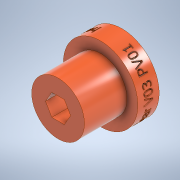
# Autodesk Inventor part: hexBushingForSideWormGear
Saved by Autodesk Inventor 2022.2 (Build 262287010, 287A)
## iProperties
Created: 2020-11-16
Part Number: hexBushingForSideWormGear
Material: PC/ABS Plastic
Document SubType Name: Modeling
Designer: robst
Density: 0.357273 g/cm^3
Appearance: Smooth - Light Orange
Author: robst
Autodesk Inventor part; units mm, degrees
ref_plane "YZ Plane" through (0, 0, 0) normal (1, 0, 0) x (0, 1, 0)
ref_plane "XY Plane" through (0, 0, 0) normal (0, 0, 1) x (1, 0, 0)
sketch "Sketch1" plane through (0, 0, 0) normal (0, 0, 1) x (1, 0, 0)
  line L0 (7.3323, 0) -> (3.6662, -6.35)
  line L1 (3.6662, -6.35) -> (-3.6662, -6.35)
  line L2 (-3.6662, -6.35) -> (-7.3323, 0)
  line L3 (-7.3323, 0) -> (-3.6662, 6.35)
  line L4 (-3.6662, 6.35) -> (3.6662, 6.35)
  line L5 (3.6662, 6.35) -> (7.3323, 0)
  point P0 (0, 0)
  point P1 (0, 0)
  dimension "d0" = 12.7
  constraints: 12 end point, 1 coincident, 1 horizontal, 13 other
  measures "d0" distance between parallel lines of L1 L4
extrude "Extrusion1" add sketch "Sketch1" along normal mid plane 25.4
sketch "Sketch2" plane through (0, 0, -12.7) normal (0, 0, -1) x (-1, 0, 0)
  circle A0 centre (0, 0) radius 15.748
  dimension "d3" = 31.496
  constraints: 1 centre point, 1 coincident
  measures "d3" diameter of A0
extrude "Extrusion2" add sketch "Sketch2" along normal blind 19.05
sketch "Sketch3" plane through (0, 0, -31.75) normal (0, 0, -1) x (-1, 0, 0)
  circle A0 centre (0, 0) radius 22.225
  dimension "d6" = 44.45
  constraints: 1 centre point, 1 coincident
  measures "d6" diameter of A0
extrude "Base" add sketch "Sketch3" along normal blind 12.7
sketch "Sketch6" plane through (-3.6662, 6.35, 12.7) normal (0, 1, 0) x (1, 0, 0)
  line L0 (7.3323, 0) -> (0, 0) construction
  line L1 (3.6662, 0) -> (3.6662, 34.6111) construction
  line L2 (19.4142, 25.4) -> (-12.0818, 25.4) projected
  point P0 (3.6662, 12.7)
  point P1 (3.6662, 19.2024)
  dimension "d13" = 6.1976
  constraints: 2 end point, 1 midpoint, 1 point on line, 1 vertical
  measures "d13" distance from line of point (3.666, 19.202) L2
hole "Hole1" at (0, 6.35, -6.5024) direction (0, -1, 0) diameter 4.318 end through all clearance for "Hex Machine Screw" size "#6" standard "Ansi Unified Screw Threads"
sketch "Sketch7" plane through (0, 0, 12.7) normal (0, 0, 1) x (1, 0, 0)
  point P0 (0, 0)
  point P1 (0, 0)
  constraints: 1 coincident
hole "Hole2" at (0, 0, 12.7) direction (0, 0, -1) diameter 6.3246 depth 7.874 counterbore diameter 6.604 counterbore depth 6.1239
ref_plane "Work Plane1" through (0, -22.225, -31.75) normal (0, 1, 0) x (-1, 0, 0)
sketch "Sketch8" plane through (0, -22.225, -31.75) normal (0, 1, 0) x (-1, 0, 0)
  line L0 (-22.225, -12.7) -> (22.225, -12.7) projected
  line L1 (-22.225, 0) -> (22.225, 0) projected
  line L2 (22.225, 0) -> (22.225, -12.7) construction
  line L3 (22.225, -6.35) -> (-22.225, -6.35) construction
  line L4 (-22.225, 0) -> (-22.225, -12.7) construction
  line L5 (58.138, -8.89) -> (58.7802, -8.89)
  line L6 (58.7802, -8.89) -> (58.7802, -6.7164)
  spline S0 degree 2 poles (58.7802, -6.7164) (58.7802, -6.4529) (58.8296, -6.0001) (58.9037, -5.8642) knots 0 0 0 1 2 2 2
  spline S1 degree 2 poles (58.9037, -5.8642) (58.9819, -5.7201) (59.2619, -5.5802) (59.5006, -5.5802) knots 0 0 0 1 2 2 2
  spline S2 degree 2 poles (59.5006, -5.5802) (59.7394, -5.5802) (60.2458, -5.8354) (60.4886, -6.0412) knots 0 0 0 1 2 2 2
  line L7 (60.4886, -6.0412) -> (60.4886, -8.89)
  line L8 (60.4886, -8.89) -> (61.1308, -8.89)
  line L9 (61.1308, -8.89) -> (61.1308, -3.5836)
  line L10 (61.1308, -3.5836) -> (60.4886, -3.5836)
  line L11 (60.4886, -3.5836) -> (60.4886, -5.502)
  spline S3 degree 2 poles (60.4886, -5.502) (60.2005, -5.2426) (59.6447, -4.9709) (59.3318, -4.9709) knots 0 0 0 1 2 2 2
  spline S4 degree 2 poles (59.3318, -4.9709) (58.772, -4.9709) (58.138, -5.7119) (58.138, -6.4159) knots 0 0 0 1 2 2 2
  line L12 (58.138, -6.4159) -> (58.138, -8.89)
  spline S5 degree 2 poles (55.5815, -8.9765) (56.4954, -8.9765) (57.4999, -7.9514) (57.4999, -7.0046) knots 0 0 0 1 2 2 2
  spline S6 degree 2 poles (57.4999, -7.0046) (57.4999, -6.0742) (56.5243, -4.9709) (55.738, -4.9709) knots 0 0 0 1 2 2 2
  spline S7 degree 2 poles (55.738, -4.9709) (55.3839, -4.9709) (54.8364, -5.1767) (54.6347, -5.3949) knots 0 0 0 1 2 2 2
  spline S8 degree 2 poles (54.6347, -5.3949) (54.4289, -5.6131) (54.2107, -6.243) (54.2107, -6.6999) knots 0 0 0 1 2 2 2
  line L13 (54.2107, -6.6999) -> (54.2107, -7.0498)
  line L14 (54.2107, -7.0498) -> (56.8495, -7.0498)
  spline S9 degree 2 poles (56.8495, -7.0498) (56.8495, -7.7126) (56.1826, -8.4166) (55.5898, -8.4166) knots 0 0 0 1 2 2 2
  spline S10 degree 2 poles (55.5898, -8.4166) (55.3798, -8.4166) (54.9723, -8.3219) (54.8076, -8.2478) knots 0 0 0 1 2 2 2
  spline S11 degree 2 poles (54.8076, -8.2478) (54.6347, -8.1655) (54.3959, -8.0214) (54.3177, -7.9555) knots 0 0 0 1 2 2 2
  line L15 (54.3177, -7.9555) -> (54.2807, -7.9555)
  line L16 (54.2807, -7.9555) -> (54.2807, -8.6553)
  spline S12 degree 2 poles (54.2807, -8.6553) (54.3918, -8.7006) (54.7294, -8.8324) (54.8611, -8.8694) knots 0 0 0 1 2 2 2
  spline S13 degree 2 poles (54.8611, -8.8694) (55.0464, -8.9229) (55.351, -8.9765) (55.5815, -8.9765) knots 0 0 0 1 2 2 2
  spline S14 degree 2 poles (54.8364, -6.56) (54.8447, -6.3006) (54.9517, -5.9219) (55.0546, -5.7942) knots 0 0 0 1 2 2 2
  spline S15 degree 2 poles (55.0546, -5.7942) (55.1658, -5.6502) (55.5157, -5.4978) (55.775, -5.4978) knots 0 0 0 1 2 2 2
  spline S16 degree 2 poles (55.775, -5.4978) (56.0303, -5.4978) (56.3884, -5.6502) (56.5366, -5.7984) knots 0 0 0 1 2 2 2
  spline S17 degree 2 poles (56.5366, -5.7984) (56.6807, -5.9507) (56.8289, -6.3171) (56.8495, -6.56) knots 0 0 0 1 2 2 2
  line L17 (56.8495, -6.56) -> (54.8364, -6.56)
  line L18 (50.6003, -8.89) -> (51.3866, -8.89)
  line L19 (51.3866, -8.89) -> (52.3129, -7.4574)
  line L20 (52.3129, -7.4574) -> (53.2638, -8.89)
  line L21 (53.2638, -8.89) -> (53.9925, -8.89)
  line L22 (53.9925, -8.89) -> (52.671, -7.0004)
  line L23 (52.671, -7.0004) -> (53.9801, -5.0779)
  line L24 (53.9801, -5.0779) -> (53.1939, -5.0779)
  line L25 (53.1939, -5.0779) -> (52.2717, -6.4982)
  line L26 (52.2717, -6.4982) -> (51.329, -5.0779)
  line L27 (51.329, -5.0779) -> (50.6003, -5.0779)
  line L28 (50.6003, -5.0779) -> (51.9136, -6.9593)
  line L29 (51.9136, -6.9593) -> (50.6003, -8.89)
  spline S18 degree 2 poles (46.6071, -7.3298) (46.6071, -7.7085) (46.8953, -8.289) (47.1341, -8.4783) knots 0 0 0 1 2 2 2
  spline S19 degree 2 poles (47.1341, -8.4783) (47.4223, -8.7006) (48.0768, -8.89) (48.5955, -8.89) knots 0 0 0 1 2 2 2
  line L30 (48.5955, -8.89) -> (50.0528, -8.89)
  line L31 (50.0528, -8.89) -> (50.0528, -3.81)
  line L32 (50.0528, -3.81) -> (48.7067, -3.81)
  spline S20 degree 2 poles (48.7067, -3.81) (48.1633, -3.81) (47.6199, -3.88) (47.3729, -4.0158) knots 0 0 0 1 2 2 2
  spline S21 degree 2 poles (47.3729, -4.0158) (47.097, -4.1599) (46.8459, -4.6333) (46.8459, -4.9544) knots 0 0 0 1 2 2 2
  spline S22 degree 2 poles (46.8459, -4.9544) (46.8459, -5.3126) (47.2247, -5.8807) (47.5581, -6.0412) knots 0 0 0 1 2 2 2
  line L33 (47.5581, -6.0412) -> (47.5581, -6.0659)
  spline S23 degree 2 poles (47.5581, -6.0659) (47.1053, -6.1894) (46.6071, -6.844) (46.6071, -7.3298) knots 0 0 0 1 2 2 2
  spline S24 degree 2 poles (47.3111, -7.3586) (47.3111, -7.0704) (47.4758, -6.6999) (47.7228, -6.5682) knots 0 0 0 1 2 2 2
  spline S25 degree 2 poles (47.7228, -6.5682) (47.8833, -6.4859) (48.2621, -6.4365) (48.612, -6.4365) knots 0 0 0 1 2 2 2
  line L34 (48.612, -6.4365) -> (49.3777, -6.4365)
  line L35 (49.3777, -6.4365) -> (49.3777, -8.3137)
  line L36 (49.3777, -8.3137) -> (48.8302, -8.3137)
  spline S26 degree 2 poles (48.8302, -8.3137) (48.3856, -8.3137) (47.8751, -8.2313) (47.6775, -8.0996) knots 0 0 0 1 2 2 2
  spline S27 degree 2 poles (47.6775, -8.0996) (47.4881, -7.9637) (47.3111, -7.6262) (47.3111, -7.3586) knots 0 0 0 1 2 2 2
  spline S28 degree 2 poles (47.5499, -5.0491) (47.5499, -4.868) (47.6734, -4.5963) (47.8092, -4.5181) knots 0 0 0 1 2 2 2
  spline S29 degree 2 poles (47.8092, -4.5181) (47.9739, -4.4275) (48.3732, -4.3863) (48.7314, -4.3863) knots 0 0 0 1 2 2 2
  line L37 (48.7314, -4.3863) -> (49.3777, -4.3863)
  line L38 (49.3777, -4.3863) -> (49.3777, -5.8725)
  line L39 (49.3777, -5.8725) -> (48.612, -5.8725)
  spline S30 degree 2 poles (48.612, -5.8725) (48.295, -5.8725) (47.9945, -5.8066) (47.8339, -5.7037) knots 0 0 0 1 2 2 2
  spline S31 degree 2 poles (47.8339, -5.7037) (47.6775, -5.6049) (47.5499, -5.2879) (47.5499, -5.0491) knots 0 0 0 1 2 2 2
  line L40 (43.0215, -8.89) -> (43.6637, -8.89)
  line L41 (43.6637, -8.89) -> (43.6637, -8.4701)
  spline S32 degree 2 poles (43.6637, -8.4701) (43.9601, -8.7294) (44.4912, -8.997) (44.8205, -8.997) knots 0 0 0 1 2 2 2
  spline S33 degree 2 poles (44.8205, -8.997) (45.0675, -8.997) (45.508, -8.8324) (45.6685, -8.6553) knots 0 0 0 1 2 2 2
  spline S34 degree 2 poles (45.6685, -8.6553) (45.8332, -8.4783) (46.0143, -7.939) (46.0143, -7.5521) knots 0 0 0 1 2 2 2
  line L42 (46.0143, -7.5521) -> (46.0143, -5.0779)
  line L43 (46.0143, -5.0779) -> (45.3721, -5.0779)
  line L44 (45.3721, -5.0779) -> (45.3721, -7.2516)
  spline S35 degree 2 poles (45.3721, -7.2516) (45.3721, -7.5562) (45.3269, -7.9555) (45.2486, -8.1037) knots 0 0 0 1 2 2 2
  spline S36 degree 2 poles (45.2486, -8.1037) (45.1704, -8.2519) (44.9028, -8.3878) (44.6517, -8.3878) knots 0 0 0 1 2 2 2
  spline S37 degree 2 poles (44.6517, -8.3878) (44.4171, -8.3878) (43.886, -8.1202) (43.6637, -7.9267) knots 0 0 0 1 2 2 2
  line L45 (43.6637, -7.9267) -> (43.6637, -5.0779)
  line L46 (43.6637, -5.0779) -> (43.0215, -5.0779)
  line L47 (43.0215, -5.0779) -> (43.0215, -8.89)
  spline S38 degree 2 poles (41.062, -8.9806) (41.4448, -8.9806) (42.1076, -8.7747) (42.3258, -8.6595) knots 0 0 0 1 2 2 2
  line L48 (42.3258, -8.6595) -> (42.3258, -7.939)
  line L49 (42.3258, -7.939) -> (42.2929, -7.939)
  spline S39 degree 2 poles (42.2929, -7.939) (42.2105, -8.0049) (41.9882, -8.1613) (41.803, -8.2478) knots 0 0 0 1 2 2 2
  spline S40 degree 2 poles (41.803, -8.2478) (41.6424, -8.326) (41.2472, -8.4413) (41.0373, -8.4413) knots 0 0 0 1 2 2 2
  spline S41 degree 2 poles (41.0373, -8.4413) (40.8849, -8.4413) (40.535, -8.3713) (40.4527, -8.3137) knots 0 0 0 1 2 2 2
  spline S42 degree 2 poles (40.4527, -8.3137) (40.3333, -8.2354) (40.2263, -8.0584) (40.2263, -7.8773) knots 0 0 0 1 2 2 2
  spline S43 degree 2 poles (40.2263, -7.8773) (40.2263, -7.6509) (40.4733, -7.4162) (40.7903, -7.338) knots 0 0 0 1 2 2 2
  spline S44 degree 2 poles (40.7903, -7.338) (40.9138, -7.3092) (41.309, -7.2269) (41.4777, -7.1816) knots 0 0 0 1 2 2 2
  spline S45 degree 2 poles (41.4777, -7.1816) (41.9141, -7.054) (42.3093, -6.527) (42.3093, -6.1524) knots 0 0 0 1 2 2 2
  spline S46 degree 2 poles (42.3093, -6.1524) (42.3093, -5.6337) (41.5313, -4.9874) (40.8891, -4.9874) knots 0 0 0 1 2 2 2
  spline S47 degree 2 poles (40.8891, -4.9874) (40.5721, -4.9874) (39.9299, -5.1438) (39.7117, -5.2632) knots 0 0 0 1 2 2 2
  line L50 (39.7117, -5.2632) -> (39.7117, -5.9507)
  line L51 (39.7117, -5.9507) -> (39.7446, -5.9507)
  spline S48 degree 2 poles (39.7446, -5.9507) (39.9916, -5.7531) (40.5927, -5.5267) (40.9014, -5.5267) knots 0 0 0 1 2 2 2
  spline S49 degree 2 poles (40.9014, -5.5267) (41.2184, -5.5267) (41.6548, -5.7942) (41.6548, -6.0618) knots 0 0 0 1 2 2 2
  spline S50 degree 2 poles (41.6548, -6.0618) (41.6548, -6.3047) (41.3954, -6.5394) (41.1072, -6.6135) knots 0 0 0 1 2 2 2
  spline S51 degree 2 poles (41.1072, -6.6135) (40.9673, -6.6505) (40.6132, -6.7246) (40.4198, -6.7699) knots 0 0 0 1 2 2 2
  spline S52 degree 2 poles (40.4198, -6.7699) (39.9999, -6.8769) (39.5717, -7.3668) (39.5717, -7.7908) knots 0 0 0 1 2 2 2
  spline S53 degree 2 poles (39.5717, -7.7908) (39.5717, -8.0378) (39.7652, -8.4742) (39.9546, -8.6348) knots 0 0 0 1 2 2 2
  spline S54 degree 2 poles (39.9546, -8.6348) (40.1563, -8.8035) (40.6709, -8.9806) (41.062, -8.9806) knots 0 0 0 1 2 2 2
  line L52 (35.982, -8.89) -> (36.6242, -8.89)
  line L53 (36.6242, -8.89) -> (36.6242, -6.7164)
  spline S55 degree 2 poles (36.6242, -6.7164) (36.6242, -6.4529) (36.6736, -6.0001) (36.7477, -5.8642) knots 0 0 0 1 2 2 2
  spline S56 degree 2 poles (36.7477, -5.8642) (36.8259, -5.7201) (37.1058, -5.5802) (37.3446, -5.5802) knots 0 0 0 1 2 2 2
  spline S57 degree 2 poles (37.3446, -5.5802) (37.5834, -5.5802) (38.0897, -5.8354) (38.3326, -6.0412) knots 0 0 0 1 2 2 2
  line L54 (38.3326, -6.0412) -> (38.3326, -8.89)
  line L55 (38.3326, -8.89) -> (38.9748, -8.89)
  line L56 (38.9748, -8.89) -> (38.9748, -3.5836)
  line L57 (38.9748, -3.5836) -> (38.3326, -3.5836)
  line L58 (38.3326, -3.5836) -> (38.3326, -5.502)
  spline S58 degree 2 poles (38.3326, -5.502) (38.0444, -5.2426) (37.4887, -4.9709) (37.1758, -4.9709) knots 0 0 0 1 2 2 2
  spline S59 degree 2 poles (37.1758, -4.9709) (36.6159, -4.9709) (35.982, -5.7119) (35.982, -6.4159) knots 0 0 0 1 2 2 2
  line L59 (35.982, -6.4159) -> (35.982, -8.89)
  line L60 (34.4259, -8.89) -> (35.0681, -8.89)
  line L61 (35.0681, -8.89) -> (35.0681, -5.0779)
  line L62 (35.0681, -5.0779) -> (34.4259, -5.0779)
  line L63 (34.4259, -5.0779) -> (34.4259, -8.89)
  line L64 (34.3806, -4.444) -> (35.1092, -4.444)
  line L65 (35.1092, -4.444) -> (35.1092, -3.7771)
  line L66 (35.1092, -3.7771) -> (34.3806, -3.7771)
  line L67 (34.3806, -3.7771) -> (34.3806, -4.444)
  line L68 (30.4903, -8.89) -> (31.1325, -8.89)
  line L69 (31.1325, -8.89) -> (31.1325, -6.7164)
  spline S60 degree 2 poles (31.1325, -6.7164) (31.1325, -6.4529) (31.1819, -6.0001) (31.256, -5.8642) knots 0 0 0 1 2 2 2
  spline S61 degree 2 poles (31.256, -5.8642) (31.3342, -5.7201) (31.6142, -5.5802) (31.8529, -5.5802) knots 0 0 0 1 2 2 2
  spline S62 degree 2 poles (31.8529, -5.5802) (32.0917, -5.5802) (32.598, -5.8354) (32.8409, -6.0412) knots 0 0 0 1 2 2 2
  line L70 (32.8409, -6.0412) -> (32.8409, -8.89)
  line L71 (32.8409, -8.89) -> (33.4831, -8.89)
  line L72 (33.4831, -8.89) -> (33.4831, -5.0779)
  line L73 (33.4831, -5.0779) -> (32.8409, -5.0779)
  line L74 (32.8409, -5.0779) -> (32.8409, -5.502)
  spline S63 degree 2 poles (32.8409, -5.502) (32.5528, -5.2426) (31.997, -4.9709) (31.6841, -4.9709) knots 0 0 0 1 2 2 2
  spline S64 degree 2 poles (31.6841, -4.9709) (31.1243, -4.9709) (30.4903, -5.7119) (30.4903, -6.4159) knots 0 0 0 1 2 2 2
  line L75 (30.4903, -6.4159) -> (30.4903, -8.89)
  spline S65 degree 2 poles (29.4529, -9.4993) (29.387, -9.5281) (29.1359, -9.6187) (28.9753, -9.6557) knots 0 0 0 1 2 2 2
  spline S66 degree 2 poles (28.9753, -9.6557) (28.7983, -9.701) (28.4978, -9.7545) (28.3208, -9.7545) knots 0 0 0 1 2 2 2
  spline S67 degree 2 poles (28.3208, -9.7545) (28.0244, -9.7545) (27.6127, -9.5981) (27.4975, -9.4581) knots 0 0 0 1 2 2 2
  spline S68 degree 2 poles (27.4975, -9.4581) (27.3863, -9.3181) (27.2999, -8.9518) (27.2999, -8.7171) knots 0 0 0 1 2 2 2
  line L76 (27.2999, -8.7171) -> (27.2999, -8.3836)
  spline S69 degree 2 poles (27.2999, -8.3836) (27.5592, -8.6101) (28.0573, -8.8241) (28.4319, -8.8241) knots 0 0 0 1 2 2 2
  spline S70 degree 2 poles (28.4319, -8.8241) (29.0824, -8.8241) (29.8522, -7.8567) (29.8522, -6.9469) knots 0 0 0 1 2 2 2
  spline S71 degree 2 poles (29.8522, -6.9469) (29.8522, -6.4735) (29.5846, -5.7407) (29.3623, -5.4814) knots 0 0 0 1 2 2 2
  spline S72 degree 2 poles (29.3623, -5.4814) (29.1483, -5.2385) (28.5596, -4.9709) (28.2467, -4.9709) knots 0 0 0 1 2 2 2
  spline S73 degree 2 poles (28.2467, -4.9709) (27.9503, -4.9709) (27.518, -5.1109) (27.2999, -5.2385) knots 0 0 0 1 2 2 2
  line L77 (27.2999, -5.2385) -> (27.2628, -5.0779)
  line L78 (27.2628, -5.0779) -> (26.6577, -5.0779)
  line L79 (26.6577, -5.0779) -> (26.6577, -8.4536)
  spline S74 degree 2 poles (26.6577, -8.4536) (26.6577, -9.4252) (27.5016, -10.3308) (28.3702, -10.3308) knots 0 0 0 1 2 2 2
  spline S75 degree 2 poles (28.3702, -10.3308) (28.6501, -10.3308) (29.2347, -10.2403) (29.4858, -10.1662) knots 0 0 0 1 2 2 2
  line L80 (29.4858, -10.1662) -> (29.4858, -9.4993)
  line L81 (29.4858, -9.4993) -> (29.4529, -9.4993)
  line L82 (27.2999, -7.8567) -> (27.2999, -5.7613)
  spline S76 degree 2 poles (27.2999, -5.7613) (27.5386, -5.646) (27.9421, -5.5472) (28.1438, -5.5472) knots 0 0 0 1 2 2 2
  spline S77 degree 2 poles (28.1438, -5.5472) (28.6295, -5.5472) (29.1894, -6.2635) (29.1894, -6.9346) knots 0 0 0 1 2 2 2
  spline S78 degree 2 poles (29.1894, -6.9346) (29.1894, -7.5685) (28.7654, -8.2313) (28.2879, -8.2313) knots 0 0 0 1 2 2 2
  spline S79 degree 2 poles (28.2879, -8.2313) (28.0367, -8.2313) (27.5098, -8.0337) (27.2999, -7.8567) knots 0 0 0 1 2 2 2
  line L83 (22.6398, -4.411) -> (25.0027, -4.411)
  line L84 (25.0027, -4.411) -> (25.0027, -5.8436)
  line L85 (25.0027, -5.8436) -> (22.7386, -5.8436)
  line L86 (22.7386, -5.8436) -> (22.7386, -6.4447)
  line L87 (22.7386, -6.4447) -> (25.0027, -6.4447)
  line L88 (25.0027, -6.4447) -> (25.0027, -8.89)
  line L89 (25.0027, -8.89) -> (25.6779, -8.89)
  line L90 (25.6779, -8.89) -> (25.6779, -3.81)
  line L91 (25.6779, -3.81) -> (22.6398, -3.81)
  line L92 (22.6398, -3.81) -> (22.6398, -4.411)
  spline S80 degree 2 poles (18.9512, -6.984) (18.9512, -7.9473) (19.8775, -8.997) (20.6514, -8.997) knots 0 0 0 1 2 2 2
  spline S81 degree 2 poles (20.6514, -8.997) (21.4459, -8.997) (22.3557, -7.9143) (22.3557, -6.984) knots 0 0 0 1 2 2 2
  spline S82 degree 2 poles (22.3557, -6.984) (22.3557, -6.0289) (21.4171, -4.9709) (20.6514, -4.9709) knots 0 0 0 1 2 2 2
  spline S83 degree 2 poles (20.6514, -4.9709) (19.8775, -4.9709) (18.9512, -6.0248) (18.9512, -6.984) knots 0 0 0 1 2 2 2
  spline S84 degree 2 poles (19.614, -6.984) (19.614, -6.243) (20.1533, -5.5225) (20.6514, -5.5225) knots 0 0 0 1 2 2 2
  spline S85 degree 2 poles (20.6514, -5.5225) (21.1495, -5.5225) (21.6929, -6.243) (21.6929, -6.984) knots 0 0 0 1 2 2 2
  spline S86 degree 2 poles (21.6929, -6.984) (21.6929, -7.7044) (21.1495, -8.4454) (20.6514, -8.4454) knots 0 0 0 1 2 2 2
  spline S87 degree 2 poles (20.6514, -8.4454) (20.1574, -8.4454) (19.614, -7.7167) (19.614, -6.984) knots 0 0 0 1 2 2 2
  line L93 (16.2712, -5.7654) -> (16.3042, -5.7654)
  spline S88 degree 2 poles (16.3042, -5.7654) (16.3783, -5.7448) (16.5388, -5.7366) (16.65, -5.7366) knots 0 0 0 1 2 2 2
  spline S89 degree 2 poles (16.65, -5.7366) (16.9093, -5.7366) (17.4198, -5.963) (17.6503, -6.1853) knots 0 0 0 1 2 2 2
  line L94 (17.6503, -6.1853) -> (17.6503, -8.89)
  line L95 (17.6503, -8.89) -> (18.2925, -8.89)
  line L96 (18.2925, -8.89) -> (18.2925, -5.0779)
  line L97 (18.2925, -5.0779) -> (17.6503, -5.0779)
  line L98 (17.6503, -5.0779) -> (17.6503, -5.646)
  spline S90 degree 2 poles (17.6503, -5.646) (17.3004, -5.3332) (16.7776, -5.0779) (16.5306, -5.0779) knots 0 0 0 1 2 2 2
  spline S91 degree 2 poles (16.5306, -5.0779) (16.4318, -5.0779) (16.333, -5.0862) (16.2712, -5.0985) knots 0 0 0 1 2 2 2
  line L99 (16.2712, -5.0985) -> (16.2712, -5.7654)
  spline S92 degree 2 poles (14.3076, -8.9806) (14.8592, -8.9806) (15.6331, -8.75) (15.9748, -8.5854) knots 0 0 0 1 2 2 2
  line L100 (15.9748, -8.5854) -> (15.9748, -7.7373)
  line L101 (15.9748, -7.7373) -> (15.9254, -7.7373)
  spline S93 degree 2 poles (15.9254, -7.7373) (15.592, -8.0502) (14.7481, -8.396) (14.357, -8.396) knots 0 0 0 1 2 2 2
  spline S94 degree 2 poles (14.357, -8.396) (13.7971, -8.396) (13.2249, -7.9308) (13.2249, -7.548) knots 0 0 0 1 2 2 2
  spline S95 degree 2 poles (13.2249, -7.548) (13.2249, -7.2433) (13.5254, -6.8646) (13.8506, -6.7699) knots 0 0 0 1 2 2 2
  spline S96 degree 2 poles (13.8506, -6.7699) (14.0853, -6.704) (14.4764, -6.6135) (14.7686, -6.5394) knots 0 0 0 1 2 2 2
  spline S97 degree 2 poles (14.7686, -6.5394) (15.0321, -6.4694) (15.4479, -6.2594) (15.6084, -6.0906) knots 0 0 0 1 2 2 2
  spline S98 degree 2 poles (15.6084, -6.0906) (15.7649, -5.9219) (15.9378, -5.469) (15.9378, -5.1726) knots 0 0 0 1 2 2 2
  spline S99 degree 2 poles (15.9378, -5.1726) (15.9378, -4.5551) (14.9745, -3.7194) (14.2294, -3.7194) knots 0 0 0 1 2 2 2
  spline S100 degree 2 poles (14.2294, -3.7194) (13.8012, -3.7194) (13.0437, -3.8882) (12.7185, -4.0488) knots 0 0 0 1 2 2 2
  line L102 (12.7185, -4.0488) -> (12.7185, -4.8556)
  line L103 (12.7185, -4.8556) -> (12.7679, -4.8556)
  spline S101 degree 2 poles (12.7679, -4.8556) (13.0108, -4.6333) (13.7683, -4.304) (14.1841, -4.304) knots 0 0 0 1 2 2 2
  spline S102 degree 2 poles (14.1841, -4.304) (14.6534, -4.304) (15.2338, -4.7445) (15.2338, -5.1026) knots 0 0 0 1 2 2 2
  spline S103 degree 2 poles (15.2338, -5.1026) (15.2338, -5.4237) (14.8921, -5.8066) (14.571, -5.893) knots 0 0 0 1 2 2 2
  spline S104 degree 2 poles (14.571, -5.893) (14.357, -5.9507) (13.7353, -6.0989) (13.5295, -6.1606) knots 0 0 0 1 2 2 2
  spline S105 degree 2 poles (13.5295, -6.1606) (13.0067, -6.3212) (12.5209, -6.9675) (12.5209, -7.4409) knots 0 0 0 1 2 2 2
  spline S106 degree 2 poles (12.5209, -7.4409) (12.5209, -7.7414) (12.7638, -8.3178) (12.982, -8.5195) knots 0 0 0 1 2 2 2
  spline S107 degree 2 poles (12.982, -8.5195) (13.2249, -8.7418) (13.8424, -8.9806) (14.3076, -8.9806) knots 0 0 0 1 2 2 2
  line L104 (11.2283, -8.89) -> (11.8705, -8.89)
  line L105 (11.8705, -8.89) -> (11.8705, -5.0779)
  line L106 (11.8705, -5.0779) -> (11.2283, -5.0779)
  line L107 (11.2283, -5.0779) -> (11.2283, -8.89)
  line L108 (11.183, -4.444) -> (11.9117, -4.444)
  line L109 (11.9117, -4.444) -> (11.9117, -3.7771)
  line L110 (11.9117, -3.7771) -> (11.183, -3.7771)
  line L111 (11.183, -3.7771) -> (11.183, -4.444)
  line L112 (7.3545, -8.89) -> (7.9967, -8.89)
  line L113 (7.9967, -8.89) -> (7.9967, -8.503)
  spline S108 degree 2 poles (7.9967, -8.503) (8.1449, -8.6265) (8.3631, -8.7912) (8.5113, -8.8612) knots 0 0 0 1 2 2 2
  spline S109 degree 2 poles (8.5113, -8.8612) (8.6471, -8.9271) (8.9394, -8.997) (9.1329, -8.997) knots 0 0 0 1 2 2 2
  spline S110 degree 2 poles (9.1329, -8.997) (9.4458, -8.997) (9.9727, -8.7377) (10.1579, -8.4866) knots 0 0 0 1 2 2 2
  spline S111 degree 2 poles (10.1579, -8.4866) (10.3432, -8.2354) (10.549, -7.4944) (10.549, -7.0128) knots 0 0 0 1 2 2 2
  spline S112 degree 2 poles (10.549, -7.0128) (10.549, -6.5106) (10.2897, -5.7778) (10.0633, -5.502) knots 0 0 0 1 2 2 2
  spline S113 degree 2 poles (10.0633, -5.502) (9.8533, -5.255) (9.2646, -4.9709) (8.9394, -4.9709) knots 0 0 0 1 2 2 2
  spline S114 degree 2 poles (8.9394, -4.9709) (8.6553, -4.9709) (8.2313, -5.0985) (7.9967, -5.2303) knots 0 0 0 1 2 2 2
  line L114 (7.9967, -5.2303) -> (7.9967, -3.5836)
  line L115 (7.9967, -3.5836) -> (7.3545, -3.5836)
  line L116 (7.3545, -3.5836) -> (7.3545, -8.89)
  line L117 (7.9967, -7.9637) -> (7.9967, -5.7613)
  spline S115 degree 2 poles (7.9967, -5.7613) (8.2354, -5.646) (8.6142, -5.5596) (8.8324, -5.5596) knots 0 0 0 1 2 2 2
  spline S116 degree 2 poles (8.8324, -5.5596) (9.3264, -5.5596) (9.8862, -6.3006) (9.8862, -7.0004) knots 0 0 0 1 2 2 2
  spline S117 degree 2 poles (9.8862, -7.0004) (9.8862, -7.6756) (9.4581, -8.3878) (8.9847, -8.3878) knots 0 0 0 1 2 2 2
  spline S118 degree 2 poles (8.9847, -8.3878) (8.7336, -8.3878) (8.2231, -8.1572) (7.9967, -7.9637) knots 0 0 0 1 2 2 2
  spline S119 degree 2 poles (4.7692, -8.9765) (5.6831, -8.9765) (6.6876, -7.9514) (6.6876, -7.0046) knots 0 0 0 1 2 2 2
  spline S120 degree 2 poles (6.6876, -7.0046) (6.6876, -6.0742) (5.7119, -4.9709) (4.9256, -4.9709) knots 0 0 0 1 2 2 2
  spline S121 degree 2 poles (4.9256, -4.9709) (4.5716, -4.9709) (4.0241, -5.1767) (3.8224, -5.3949) knots 0 0 0 1 2 2 2
  spline S122 degree 2 poles (3.8224, -5.3949) (3.6165, -5.6131) (3.3983, -6.243) (3.3983, -6.6999) knots 0 0 0 1 2 2 2
  line L118 (3.3983, -6.6999) -> (3.3983, -7.0498)
  line L119 (3.3983, -7.0498) -> (6.0371, -7.0498)
  spline S123 degree 2 poles (6.0371, -7.0498) (6.0371, -7.7126) (5.3702, -8.4166) (4.7774, -8.4166) knots 0 0 0 1 2 2 2
  spline S124 degree 2 poles (4.7774, -8.4166) (4.5675, -8.4166) (4.1599, -8.3219) (3.9953, -8.2478) knots 0 0 0 1 2 2 2
  spline S125 degree 2 poles (3.9953, -8.2478) (3.8224, -8.1655) (3.5836, -8.0214) (3.5054, -7.9555) knots 0 0 0 1 2 2 2
  line L120 (3.5054, -7.9555) -> (3.4683, -7.9555)
  line L121 (3.4683, -7.9555) -> (3.4683, -8.6553)
  spline S126 degree 2 poles (3.4683, -8.6553) (3.5795, -8.7006) (3.917, -8.8324) (4.0488, -8.8694) knots 0 0 0 1 2 2 2
  spline S127 degree 2 poles (4.0488, -8.8694) (4.234, -8.9229) (4.5387, -8.9765) (4.7692, -8.9765) knots 0 0 0 1 2 2 2
  spline S128 degree 2 poles (4.0241, -6.56) (4.0323, -6.3006) (4.1393, -5.9219) (4.2423, -5.7942) knots 0 0 0 1 2 2 2
  spline S129 degree 2 poles (4.2423, -5.7942) (4.3534, -5.6502) (4.7033, -5.4978) (4.9627, -5.4978) knots 0 0 0 1 2 2 2
  spline S130 degree 2 poles (4.9627, -5.4978) (5.2179, -5.4978) (5.5761, -5.6502) (5.7243, -5.7984) knots 0 0 0 1 2 2 2
  spline S131 degree 2 poles (5.7243, -5.7984) (5.8683, -5.9507) (6.0165, -6.3171) (6.0371, -6.56) knots 0 0 0 1 2 2 2
  line L122 (6.0371, -6.56) -> (4.0241, -6.56)
  line L123 (-2.9949, -3.81) -> (-1.7187, -8.89)
  line L124 (-1.7187, -8.89) -> (-0.9612, -8.89)
  line L125 (-0.9612, -8.89) -> (0.072, -4.6745)
  line L126 (0.072, -4.6745) -> (1.0765, -8.89)
  line L127 (1.0765, -8.89) -> (1.8258, -8.89)
  line L128 (1.8258, -8.89) -> (3.1225, -3.81)
  line L129 (3.1225, -3.81) -> (2.4268, -3.81)
  line L130 (2.4268, -3.81) -> (1.4059, -8.0214)
  line L131 (1.4059, -8.0214) -> (0.3931, -3.81)
  line L132 (0.3931, -3.81) -> (-0.2943, -3.81)
  line L133 (-0.2943, -3.81) -> (-1.3153, -8.0708)
  line L134 (-1.3153, -8.0708) -> (-2.3321, -3.81)
  line L135 (-2.3321, -3.81) -> (-2.9949, -3.81)
  spline S132 degree 2 poles (-6.6835, -6.984) (-6.6835, -7.9473) (-5.7572, -8.997) (-4.9833, -8.997) knots 0 0 0 1 2 2 2
  spline S133 degree 2 poles (-4.9833, -8.997) (-4.1887, -8.997) (-3.2789, -7.9143) (-3.2789, -6.984) knots 0 0 0 1 2 2 2
  spline S134 degree 2 poles (-3.2789, -6.984) (-3.2789, -6.0289) (-4.2176, -4.9709) (-4.9833, -4.9709) knots 0 0 0 1 2 2 2
  spline S135 degree 2 poles (-4.9833, -4.9709) (-5.7572, -4.9709) (-6.6835, -6.0248) (-6.6835, -6.984) knots 0 0 0 1 2 2 2
  spline S136 degree 2 poles (-6.0207, -6.984) (-6.0207, -6.243) (-5.4814, -5.5225) (-4.9833, -5.5225) knots 0 0 0 1 2 2 2
  spline S137 degree 2 poles (-4.9833, -5.5225) (-4.4851, -5.5225) (-3.9417, -6.243) (-3.9417, -6.984) knots 0 0 0 1 2 2 2
  spline S138 degree 2 poles (-3.9417, -6.984) (-3.9417, -7.7044) (-4.4851, -8.4454) (-4.9833, -8.4454) knots 0 0 0 1 2 2 2
  spline S139 degree 2 poles (-4.9833, -8.4454) (-5.4773, -8.4454) (-6.0207, -7.7167) (-6.0207, -6.984) knots 0 0 0 1 2 2 2
  line L136 (-9.3634, -5.7654) -> (-9.3305, -5.7654)
  spline S140 degree 2 poles (-9.3305, -5.7654) (-9.2564, -5.7448) (-9.0958, -5.7366) (-8.9847, -5.7366) knots 0 0 0 1 2 2 2
  spline S141 degree 2 poles (-8.9847, -5.7366) (-8.7253, -5.7366) (-8.2149, -5.963) (-7.9843, -6.1853) knots 0 0 0 1 2 2 2
  line L137 (-7.9843, -6.1853) -> (-7.9843, -8.89)
  line L138 (-7.9843, -8.89) -> (-7.3421, -8.89)
  line L139 (-7.3421, -8.89) -> (-7.3421, -5.0779)
  line L140 (-7.3421, -5.0779) -> (-7.9843, -5.0779)
  line L141 (-7.9843, -5.0779) -> (-7.9843, -5.646)
  spline S142 degree 2 poles (-7.9843, -5.646) (-8.3342, -5.3332) (-8.8571, -5.0779) (-9.1041, -5.0779) knots 0 0 0 1 2 2 2
  spline S143 degree 2 poles (-9.1041, -5.0779) (-9.2029, -5.0779) (-9.3017, -5.0862) (-9.3634, -5.0985) knots 0 0 0 1 2 2 2
  line L142 (-9.3634, -5.0985) -> (-9.3634, -5.7654)
  line L143 (-14.1841, -8.89) -> (-14.1841, -6.6835)
  spline S144 degree 2 poles (-14.1841, -6.6835) (-14.1841, -6.42) (-14.1429, -5.9713) (-14.077, -5.8478) knots 0 0 0 1 2 2 2
  spline S145 degree 2 poles (-14.077, -5.8478) (-14.0112, -5.7119) (-13.76, -5.5802) (-13.5419, -5.5802) knots 0 0 0 1 2 2 2
  spline S146 degree 2 poles (-13.5419, -5.5802) (-13.3443, -5.5802) (-12.8914, -5.8231) (-12.6527, -6.0536) knots 0 0 0 1 2 2 2
  spline S147 degree 2 poles (-12.6527, -6.0536) (-12.6568, -6.1112) (-12.665, -6.2718) (-12.665, -6.3788) knots 0 0 0 1 2 2 2
  line L144 (-12.665, -6.3788) -> (-12.665, -8.89)
  line L145 (-12.665, -8.89) -> (-12.0228, -8.89)
  line L146 (-12.0228, -8.89) -> (-12.0228, -6.6835)
  spline S148 degree 2 poles (-12.0228, -6.6835) (-12.0228, -6.42) (-11.9816, -5.9713) (-11.9158, -5.8478) knots 0 0 0 1 2 2 2
  spline S149 degree 2 poles (-11.9158, -5.8478) (-11.8499, -5.7119) (-11.5988, -5.5802) (-11.3806, -5.5802) knots 0 0 0 1 2 2 2
  spline S150 degree 2 poles (-11.3806, -5.5802) (-11.1748, -5.5802) (-10.7178, -5.8395) (-10.5037, -6.0412) knots 0 0 0 1 2 2 2
  line L147 (-10.5037, -6.0412) -> (-10.5037, -8.89)
  line L148 (-10.5037, -8.89) -> (-9.8615, -8.89)
  line L149 (-9.8615, -8.89) -> (-9.8615, -5.0779)
  line L150 (-9.8615, -5.0779) -> (-10.5037, -5.0779)
  line L151 (-10.5037, -5.0779) -> (-10.5037, -5.4978)
  spline S151 degree 2 poles (-10.5037, -5.4978) (-10.7549, -5.2467) (-11.2489, -4.9709) (-11.5453, -4.9709) knots 0 0 0 1 2 2 2
  spline S152 degree 2 poles (-11.5453, -4.9709) (-11.8828, -4.9709) (-12.4057, -5.2797) (-12.5415, -5.6296) knots 0 0 0 1 2 2 2
  spline S153 degree 2 poles (-12.5415, -5.6296) (-12.8338, -5.3044) (-13.3854, -4.9709) (-13.7065, -4.9709) knots 0 0 0 1 2 2 2
  spline S154 degree 2 poles (-13.7065, -4.9709) (-13.9535, -4.9709) (-14.357, -5.1232) (-14.5052, -5.2961) knots 0 0 0 1 2 2 2
  spline S155 degree 2 poles (-14.5052, -5.2961) (-14.6575, -5.469) (-14.8263, -5.9877) (-14.8263, -6.3788) knots 0 0 0 1 2 2 2
  line L152 (-14.8263, -6.3788) -> (-14.8263, -8.89)
  line L153 (-14.8263, -8.89) -> (-14.1841, -8.89)
  spline S156 degree 2 poles (-17.9056, -8.9888) (-17.3663, -8.9888) (-16.4729, -8.6595) (-16.1518, -8.326) knots 0 0 0 1 2 2 2
  spline S157 degree 2 poles (-16.1518, -8.326) (-15.8307, -7.9884) (-15.4891, -6.9922) (-15.4891, -6.3459) knots 0 0 0 1 2 2 2
  spline S158 degree 2 poles (-15.4891, -6.3459) (-15.4891, -5.7325) (-15.8349, -4.761) (-16.156, -4.4152) knots 0 0 0 1 2 2 2
  spline S159 degree 2 poles (-16.156, -4.4152) (-16.4647, -4.0817) (-17.3704, -3.7194) (-17.9097, -3.7194) knots 0 0 0 1 2 2 2
  spline S160 degree 2 poles (-17.9097, -3.7194) (-18.169, -3.7194) (-18.6383, -3.7935) (-18.8524, -3.8594) knots 0 0 0 1 2 2 2
  spline S161 degree 2 poles (-18.8524, -3.8594) (-19.0253, -3.9088) (-19.4452, -4.0899) (-19.5728, -4.1558) knots 0 0 0 1 2 2 2
  line L154 (-19.5728, -4.1558) -> (-19.5728, -4.9709)
  line L155 (-19.5728, -4.9709) -> (-19.5152, -4.9709)
  spline S162 degree 2 poles (-19.5152, -4.9709) (-19.3876, -4.8598) (-19.12, -4.658) (-18.873, -4.5428) knots 0 0 0 1 2 2 2
  spline S163 degree 2 poles (-18.873, -4.5428) (-18.6671, -4.4399) (-18.1361, -4.304) (-17.8315, -4.304) knots 0 0 0 1 2 2 2
  spline S164 degree 2 poles (-17.8315, -4.304) (-17.0987, -4.304) (-16.193, -5.4073) (-16.193, -6.3253) knots 0 0 0 1 2 2 2
  spline S165 degree 2 poles (-16.193, -6.3253) (-16.193, -6.8358) (-16.4318, -7.6015) (-16.6582, -7.8649) knots 0 0 0 1 2 2 2
  spline S166 degree 2 poles (-16.6582, -7.8649) (-16.8764, -8.1284) (-17.4939, -8.4042) (-17.8809, -8.4042) knots 0 0 0 1 2 2 2
  spline S167 degree 2 poles (-17.8809, -8.4042) (-18.1649, -8.4042) (-18.733, -8.3219) (-18.9265, -8.2396) knots 0 0 0 1 2 2 2
  line L156 (-18.9265, -8.2396) -> (-18.9265, -6.9263)
  line L157 (-18.9265, -6.9263) -> (-17.7491, -6.9263)
  line L158 (-17.7491, -6.9263) -> (-17.7491, -6.3335)
  line L159 (-17.7491, -6.3335) -> (-19.5934, -6.3335)
  line L160 (-19.5934, -6.3335) -> (-19.5934, -8.5524)
  spline S168 degree 2 poles (-19.5934, -8.5524) (-19.4658, -8.6101) (-19.0294, -8.7871) (-18.8442, -8.8406) knots 0 0 0 1 2 2 2
  spline S169 degree 2 poles (-18.8442, -8.8406) (-18.593, -8.9147) (-18.1896, -8.9888) (-17.9056, -8.9888) knots 0 0 0 1 2 2 2
  spline S170 degree 2 poles (-22.047, -8.9765) (-21.133, -8.9765) (-20.1286, -7.9514) (-20.1286, -7.0046) knots 0 0 0 1 2 2 2
  spline S171 degree 2 poles (-20.1286, -7.0046) (-20.1286, -6.0742) (-21.1042, -4.9709) (-21.8905, -4.9709) knots 0 0 0 1 2 2 2
  spline S172 degree 2 poles (-21.8905, -4.9709) (-22.2446, -4.9709) (-22.7921, -5.1767) (-22.9938, -5.3949) knots 0 0 0 1 2 2 2
  spline S173 degree 2 poles (-22.9938, -5.3949) (-23.1996, -5.6131) (-23.4178, -6.243) (-23.4178, -6.6999) knots 0 0 0 1 2 2 2
  line L161 (-23.4178, -6.6999) -> (-23.4178, -7.0498)
  line L162 (-23.4178, -7.0498) -> (-20.779, -7.0498)
  spline S174 degree 2 poles (-20.779, -7.0498) (-20.779, -7.7126) (-21.4459, -8.4166) (-22.0387, -8.4166) knots 0 0 0 1 2 2 2
  spline S175 degree 2 poles (-22.0387, -8.4166) (-22.2487, -8.4166) (-22.6562, -8.3219) (-22.8209, -8.2478) knots 0 0 0 1 2 2 2
  spline S176 degree 2 poles (-22.8209, -8.2478) (-22.9938, -8.1655) (-23.2326, -8.0214) (-23.3108, -7.9555) knots 0 0 0 1 2 2 2
  line L163 (-23.3108, -7.9555) -> (-23.3478, -7.9555)
  line L164 (-23.3478, -7.9555) -> (-23.3478, -8.6553)
  spline S177 degree 2 poles (-23.3478, -8.6553) (-23.2367, -8.7006) (-22.8991, -8.8324) (-22.7674, -8.8694) knots 0 0 0 1 2 2 2
  spline S178 degree 2 poles (-22.7674, -8.8694) (-22.5821, -8.9229) (-22.2775, -8.9765) (-22.047, -8.9765) knots 0 0 0 1 2 2 2
  spline S179 degree 2 poles (-22.7921, -6.56) (-22.7838, -6.3006) (-22.6768, -5.9219) (-22.5739, -5.7942) knots 0 0 0 1 2 2 2
  spline S180 degree 2 poles (-22.5739, -5.7942) (-22.4627, -5.6502) (-22.1128, -5.4978) (-21.8535, -5.4978) knots 0 0 0 1 2 2 2
  spline S181 degree 2 poles (-21.8535, -5.4978) (-21.5982, -5.4978) (-21.2401, -5.6502) (-21.0919, -5.7984) knots 0 0 0 1 2 2 2
  spline S182 degree 2 poles (-21.0919, -5.7984) (-20.9478, -5.9507) (-20.7996, -6.3171) (-20.779, -6.56) knots 0 0 0 1 2 2 2
  line L165 (-20.779, -6.56) -> (-22.7921, -6.56)
  spline S183 degree 2 poles (-26.1925, -8.4866) (-26.1142, -8.5442) (-25.8508, -8.75) (-25.7273, -8.8118) knots 0 0 0 1 2 2 2
  spline S184 degree 2 poles (-25.7273, -8.8118) (-25.5585, -8.9024) (-25.2415, -8.997) (-24.9533, -8.997) knots 0 0 0 1 2 2 2
  spline S185 degree 2 poles (-24.9533, -8.997) (-24.7187, -8.997) (-24.2947, -8.82) (-24.1341, -8.6595) knots 0 0 0 1 2 2 2
  spline S186 degree 2 poles (-24.1341, -8.6595) (-23.9818, -8.503) (-23.7965, -8.042) (-23.7965, -7.7867) knots 0 0 0 1 2 2 2
  spline S187 degree 2 poles (-23.7965, -7.7867) (-23.7965, -7.3915) (-24.13, -6.8317) (-24.4923, -6.6711) knots 0 0 0 1 2 2 2
  spline S188 degree 2 poles (-24.4923, -6.6711) (-24.8134, -6.5229) (-25.6861, -6.4118) (-26.1925, -6.3829) knots 0 0 0 1 2 2 2
  line L166 (-26.1925, -6.3829) -> (-26.1925, -6.2594)
  spline S189 degree 2 poles (-26.1925, -6.2594) (-26.1925, -6.0371) (-26.0566, -5.7613) (-25.9331, -5.6831) knots 0 0 0 1 2 2 2
  spline S190 degree 2 poles (-25.9331, -5.6831) (-25.8096, -5.6049) (-25.4556, -5.5555) (-25.2662, -5.5555) knots 0 0 0 1 2 2 2
  spline S191 degree 2 poles (-25.2662, -5.5555) (-25.0439, -5.5555) (-24.4429, -5.6872) (-24.1423, -5.8148) knots 0 0 0 1 2 2 2
  line L167 (-24.1423, -5.8148) -> (-24.1053, -5.8148)
  line L168 (-24.1053, -5.8148) -> (-24.1053, -5.1603)
  spline S192 degree 2 poles (-24.1053, -5.1603) (-24.2823, -5.1109) (-24.9451, -4.9874) (-25.2703, -4.9874) knots 0 0 0 1 2 2 2
  spline S193 degree 2 poles (-25.2703, -4.9874) (-25.6655, -4.9874) (-26.2048, -5.1109) (-26.4189, -5.2714) knots 0 0 0 1 2 2 2
  spline S194 degree 2 poles (-26.4189, -5.2714) (-26.6288, -5.4279) (-26.8347, -5.926) (-26.8347, -6.2841) knots 0 0 0 1 2 2 2
  line L169 (-26.8347, -6.2841) -> (-26.8347, -8.89)
  line L170 (-26.8347, -8.89) -> (-26.1925, -8.89)
  line L171 (-26.1925, -8.89) -> (-26.1925, -8.4866)
  line L172 (-26.1925, -7.9514) -> (-26.1925, -6.8934)
  spline S195 degree 2 poles (-26.1925, -6.8934) (-25.9619, -6.914) (-25.2662, -6.984) (-25.048, -7.0498) knots 0 0 0 1 2 2 2
  spline S196 degree 2 poles (-25.048, -7.0498) (-24.7928, -7.1281) (-24.4593, -7.4533) (-24.4593, -7.7414) knots 0 0 0 1 2 2 2
  spline S197 degree 2 poles (-24.4593, -7.7414) (-24.4593, -8.0708) (-24.8298, -8.4042) (-25.1839, -8.4042) knots 0 0 0 1 2 2 2
  spline S198 degree 2 poles (-25.1839, -8.4042) (-25.4844, -8.4042) (-25.9784, -8.1449) (-26.1925, -7.9514) knots 0 0 0 1 2 2 2
  line L173 (-29.7575, -5.7654) -> (-29.7246, -5.7654)
  spline S199 degree 2 poles (-29.7246, -5.7654) (-29.6505, -5.7448) (-29.4899, -5.7366) (-29.3788, -5.7366) knots 0 0 0 1 2 2 2
  spline S200 degree 2 poles (-29.3788, -5.7366) (-29.1194, -5.7366) (-28.609, -5.963) (-28.3784, -6.1853) knots 0 0 0 1 2 2 2
  line L174 (-28.3784, -6.1853) -> (-28.3784, -8.89)
  line L175 (-28.3784, -8.89) -> (-27.7362, -8.89)
  line L176 (-27.7362, -8.89) -> (-27.7362, -5.0779)
  line L177 (-27.7362, -5.0779) -> (-28.3784, -5.0779)
  line L178 (-28.3784, -5.0779) -> (-28.3784, -5.646)
  spline S201 degree 2 poles (-28.3784, -5.646) (-28.7283, -5.3332) (-29.2512, -5.0779) (-29.4982, -5.0779) knots 0 0 0 1 2 2 2
  spline S202 degree 2 poles (-29.4982, -5.0779) (-29.597, -5.0779) (-29.6958, -5.0862) (-29.7575, -5.0985) knots 0 0 0 1 2 2 2
  line L179 (-29.7575, -5.0985) -> (-29.7575, -5.7654)
  line L180 (-36.1713, -3.81) -> (-34.4217, -8.89)
  line L181 (-34.4217, -8.89) -> (-33.6931, -8.89)
  line L182 (-33.6931, -8.89) -> (-31.9435, -3.81)
  line L183 (-31.9435, -3.81) -> (-32.668, -3.81)
  line L184 (-32.668, -3.81) -> (-34.0759, -8.0296)
  line L185 (-34.0759, -8.0296) -> (-35.4838, -3.81)
  line L186 (-35.4838, -3.81) -> (-36.1713, -3.81)
  spline S203 degree 2 poles (-39.7323, -6.35) (-39.7323, -7.7167) (-38.9377, -8.997) (-38.1103, -8.997) knots 0 0 0 1 2 2 2
  spline S204 degree 2 poles (-38.1103, -8.997) (-37.2705, -8.997) (-36.4842, -7.692) (-36.4842, -6.3541) knots 0 0 0 1 2 2 2
  spline S205 degree 2 poles (-36.4842, -6.3541) (-36.4842, -4.9791) (-37.2787, -3.7071) (-38.1103, -3.7071) knots 0 0 0 1 2 2 2
  spline S206 degree 2 poles (-38.1103, -3.7071) (-38.946, -3.7071) (-39.7323, -5.0244) (-39.7323, -6.35) knots 0 0 0 1 2 2 2
  spline S207 degree 2 poles (-38.8595, -7.8979) (-38.9583, -7.6468) (-39.0407, -6.8728) (-39.0407, -6.35) knots 0 0 0 1 2 2 2
  spline S208 degree 2 poles (-39.0407, -6.35) (-39.0407, -5.8272) (-38.9583, -5.0574) (-38.8554, -4.798) knots 0 0 0 1 2 2 2
  spline S209 degree 2 poles (-38.8554, -4.798) (-38.7525, -4.5387) (-38.3943, -4.2711) (-38.1103, -4.2711) knots 0 0 0 1 2 2 2
  spline S210 degree 2 poles (-38.1103, -4.2711) (-37.8262, -4.2711) (-37.4599, -4.5387) (-37.3528, -4.8062) knots 0 0 0 1 2 2 2
  spline S211 degree 2 poles (-37.3528, -4.8062) (-37.2499, -5.0656) (-37.1758, -5.856) (-37.1758, -6.3541) knots 0 0 0 1 2 2 2
  spline S212 degree 2 poles (-37.1758, -6.3541) (-37.1758, -6.8893) (-37.2417, -7.6056) (-37.3487, -7.8855) knots 0 0 0 1 2 2 2
  spline S213 degree 2 poles (-37.3487, -7.8855) (-37.4475, -8.149) (-37.8139, -8.433) (-38.1103, -8.433) knots 0 0 0 1 2 2 2
  spline S214 degree 2 poles (-38.1103, -8.433) (-38.3902, -8.433) (-38.7566, -8.1655) (-38.8595, -7.8979) knots 0 0 0 1 2 2 2
  spline S215 degree 2 poles (-41.7536, -4.2917) (-41.5683, -4.2917) (-41.2019, -4.3822) (-41.0249, -4.4522) knots 0 0 0 1 2 2 2
  spline S216 degree 2 poles (-41.0249, -4.4522) (-40.8602, -4.5222) (-40.6174, -4.6704) (-40.5227, -4.7363) knots 0 0 0 1 2 2 2
  line L187 (-40.5227, -4.7363) -> (-40.4815, -4.7363)
  line L188 (-40.4815, -4.7363) -> (-40.4815, -4.0158)
  spline S217 degree 2 poles (-40.4815, -4.0158) (-40.7038, -3.8965) (-41.4654, -3.703) (-41.8071, -3.703) knots 0 0 0 1 2 2 2
  spline S218 degree 2 poles (-41.8071, -3.703) (-42.1529, -3.703) (-42.6675, -3.8429) (-42.8774, -3.9911) knots 0 0 0 1 2 2 2
  spline S219 degree 2 poles (-42.8774, -3.9911) (-43.0997, -4.1517) (-43.3303, -4.6169) (-43.3303, -4.9297) knots 0 0 0 1 2 2 2
  spline S220 degree 2 poles (-43.3303, -4.9297) (-43.3303, -5.3496) (-42.7786, -5.9836) (-42.3917, -6.0659) knots 0 0 0 1 2 2 2
  line L189 (-42.3917, -6.0659) -> (-42.3917, -6.1153)
  spline S221 degree 2 poles (-42.3917, -6.1153) (-42.5522, -6.1483) (-42.9186, -6.2965) (-43.075, -6.4447) knots 0 0 0 1 2 2 2
  spline S222 degree 2 poles (-43.075, -6.4447) (-43.2315, -6.5888) (-43.4291, -7.0498) (-43.4291, -7.3833) knots 0 0 0 1 2 2 2
  spline S223 degree 2 poles (-43.4291, -7.3833) (-43.4291, -7.725) (-43.1944, -8.3054) (-42.9803, -8.5277) knots 0 0 0 1 2 2 2
  spline S224 degree 2 poles (-42.9803, -8.5277) (-42.758, -8.7583) (-42.1282, -8.997) (-41.7289, -8.997) knots 0 0 0 1 2 2 2
  spline S225 degree 2 poles (-41.7289, -8.997) (-41.346, -8.997) (-40.5968, -8.8118) (-40.3415, -8.6842) knots 0 0 0 1 2 2 2
  line L190 (-40.3415, -8.6842) -> (-40.3415, -7.9637)
  line L191 (-40.3415, -7.9637) -> (-40.3909, -7.9637)
  spline S226 degree 2 poles (-40.3909, -7.9637) (-40.605, -8.1202) (-41.3295, -8.4083) (-41.6877, -8.4083) knots 0 0 0 1 2 2 2
  spline S227 degree 2 poles (-41.6877, -8.4083) (-41.8976, -8.4083) (-42.3176, -8.2766) (-42.4575, -8.1243) knots 0 0 0 1 2 2 2
  spline S228 degree 2 poles (-42.4575, -8.1243) (-42.5934, -7.972) (-42.7375, -7.6097) (-42.7375, -7.3339) knots 0 0 0 1 2 2 2
  spline S229 degree 2 poles (-42.7375, -7.3339) (-42.7375, -7.0581) (-42.5769, -6.6999) (-42.4328, -6.597) knots 0 0 0 1 2 2 2
  spline S230 degree 2 poles (-42.4328, -6.597) (-42.2887, -6.4941) (-41.8976, -6.4159) (-41.6671, -6.4159) knots 0 0 0 1 2 2 2
  line L192 (-41.6671, -6.4159) -> (-41.3789, -6.4159)
  line L193 (-41.3789, -6.4159) -> (-41.3789, -5.8519)
  line L194 (-41.3789, -5.8519) -> (-41.6054, -5.8519)
  spline S231 degree 2 poles (-41.6054, -5.8519) (-42.0623, -5.8519) (-42.6387, -5.4155) (-42.6387, -4.9997) knots 0 0 0 1 2 2 2
  spline S232 degree 2 poles (-42.6387, -4.9997) (-42.6387, -4.8062) (-42.4905, -4.5304) (-42.3711, -4.4481) knots 0 0 0 1 2 2 2
  spline S233 degree 2 poles (-42.3711, -4.4481) (-42.2435, -4.3616) (-41.9306, -4.2917) (-41.7536, -4.2917) knots 0 0 0 1 2 2 2
  spline S234 degree 2 poles (-49.7317, -5.3414) (-49.7317, -5.6707) (-49.4971, -6.2635) (-49.2871, -6.4694) knots 0 0 0 1 2 2 2
  spline S235 degree 2 poles (-49.2871, -6.4694) (-49.0236, -6.7287) (-48.3115, -6.9963) (-47.7681, -6.9963) knots 0 0 0 1 2 2 2
  line L195 (-47.7681, -6.9963) -> (-47.1958, -6.9963)
  line L196 (-47.1958, -6.9963) -> (-47.1958, -8.89)
  line L197 (-47.1958, -8.89) -> (-46.5207, -8.89)
  line L198 (-46.5207, -8.89) -> (-46.5207, -3.81)
  line L199 (-46.5207, -3.81) -> (-47.7969, -3.81)
  spline S236 degree 2 poles (-47.7969, -3.81) (-48.2497, -3.81) (-48.8837, -3.9582) (-49.1266, -4.127) knots 0 0 0 1 2 2 2
  spline S237 degree 2 poles (-49.1266, -4.127) (-49.4106, -4.3205) (-49.7317, -4.9174) (-49.7317, -5.3414) knots 0 0 0 1 2 2 2
  spline S238 degree 2 poles (-49.0278, -5.362) (-49.0278, -5.0985) (-48.8466, -4.7116) (-48.6614, -4.5881) knots 0 0 0 1 2 2 2
  spline S239 degree 2 poles (-48.6614, -4.5881) (-48.5008, -4.481) (-48.0727, -4.3946) (-47.7557, -4.3946) knots 0 0 0 1 2 2 2
  line L200 (-47.7557, -4.3946) -> (-47.1958, -4.3946)
  line L201 (-47.1958, -4.3946) -> (-47.1958, -6.42)
  line L202 (-47.1958, -6.42) -> (-47.6569, -6.42)
  spline S240 degree 2 poles (-47.6569, -6.42) (-48.0686, -6.42) (-48.5749, -6.2882) (-48.7396, -6.1153) knots 0 0 0 1 2 2 2
  spline S241 degree 2 poles (-48.7396, -6.1153) (-48.8919, -5.963) (-49.0278, -5.6049) (-49.0278, -5.362) knots 0 0 0 1 2 2 2
  line L203 (-54.0584, -3.81) -> (-52.3088, -8.89)
  line L204 (-52.3088, -8.89) -> (-51.5801, -8.89)
  line L205 (-51.5801, -8.89) -> (-49.8305, -3.81)
  line L206 (-49.8305, -3.81) -> (-50.5551, -3.81)
  line L207 (-50.5551, -3.81) -> (-51.963, -8.0296)
  line L208 (-51.963, -8.0296) -> (-53.3709, -3.81)
  line L209 (-53.3709, -3.81) -> (-54.0584, -3.81)
  spline S242 degree 2 poles (-57.6193, -6.35) (-57.6193, -7.7167) (-56.8248, -8.997) (-55.9973, -8.997) knots 0 0 0 1 2 2 2
  spline S243 degree 2 poles (-55.9973, -8.997) (-55.1575, -8.997) (-54.3712, -7.692) (-54.3712, -6.3541) knots 0 0 0 1 2 2 2
  spline S244 degree 2 poles (-54.3712, -6.3541) (-54.3712, -4.9791) (-55.1658, -3.7071) (-55.9973, -3.7071) knots 0 0 0 1 2 2 2
  spline S245 degree 2 poles (-55.9973, -3.7071) (-56.833, -3.7071) (-57.6193, -5.0244) (-57.6193, -6.35) knots 0 0 0 1 2 2 2
  spline S246 degree 2 poles (-56.7466, -7.8979) (-56.8454, -7.6468) (-56.9277, -6.8728) (-56.9277, -6.35) knots 0 0 0 1 2 2 2
  spline S247 degree 2 poles (-56.9277, -6.35) (-56.9277, -5.8272) (-56.8454, -5.0574) (-56.7424, -4.798) knots 0 0 0 1 2 2 2
  spline S248 degree 2 poles (-56.7424, -4.798) (-56.6395, -4.5387) (-56.2814, -4.2711) (-55.9973, -4.2711) knots 0 0 0 1 2 2 2
  spline S249 degree 2 poles (-55.9973, -4.2711) (-55.7133, -4.2711) (-55.3469, -4.5387) (-55.2399, -4.8062) knots 0 0 0 1 2 2 2
  spline S250 degree 2 poles (-55.2399, -4.8062) (-55.1369, -5.0656) (-55.0628, -5.856) (-55.0628, -6.3541) knots 0 0 0 1 2 2 2
  spline S251 degree 2 poles (-55.0628, -6.3541) (-55.0628, -6.8893) (-55.1287, -7.6056) (-55.2357, -7.8855) knots 0 0 0 1 2 2 2
  spline S252 degree 2 poles (-55.2357, -7.8855) (-55.3345, -8.149) (-55.7009, -8.433) (-55.9973, -8.433) knots 0 0 0 1 2 2 2
  spline S253 degree 2 poles (-55.9973, -8.433) (-56.2773, -8.433) (-56.6436, -8.1655) (-56.7466, -7.8979) knots 0 0 0 1 2 2 2
  line L210 (-61.1473, -8.89) -> (-58.6691, -8.89)
  line L211 (-58.6691, -8.89) -> (-58.6691, -8.3713)
  line L212 (-58.6691, -8.3713) -> (-59.5912, -8.3713)
  line L213 (-59.5912, -8.3713) -> (-59.5912, -4.9668)
  line L214 (-59.5912, -4.9668) -> (-58.6691, -4.9668)
  line L215 (-58.6691, -4.9668) -> (-58.6691, -4.5016)
  spline S254 degree 2 poles (-58.6691, -4.5016) (-59.1919, -4.5016) (-59.6859, -4.2052) (-59.7188, -3.7935) knots 0 0 0 1 2 2 2
  line L216 (-59.7188, -3.7935) -> (-60.2458, -3.7935)
  line L217 (-60.2458, -3.7935) -> (-60.2458, -8.3713)
  line L218 (-60.2458, -8.3713) -> (-61.1473, -8.3713)
  line L219 (-61.1473, -8.3713) -> (-61.1473, -8.89)
  point P0 (0, 31.75)
  constraints: 2 end point, 2 midpoint, 1 horizontal
emboss "Emboss2" sketch "Sketch8" operation cut depth 2.54 direction (0, -1, 0) wrap yes faces at (-22.1529, -1.7884, -40.2167)
sketch "Sketch9" plane through (0, 0, -12.7) normal (0, 0, 1) x (1, 0, 0)
  line L0 (3.6662, 6.35) -> (7.3323, 0)
  line L1 (7.3323, 0) -> (3.6662, -6.35)
  line L2 (3.6662, -6.35) -> (-3.6662, -6.35)
  line L3 (-3.6662, -6.35) -> (-7.3323, 0)
  line L4 (-7.3323, 0) -> (-3.6662, 6.35)
  line L5 (-3.6662, 6.35) -> (3.6662, 6.35)
  line L6 (3.6662, 6.35) -> (-3.6662, 6.35) projected
  point P0 (0, 0)
  point P1 (0, 0)
  constraints: 12 end point, 1 coincident, 1 collinear, 13 other
extrude "Extrusion4" cut sketch "Sketch9" along normal blind 25.4
sketch "Sketch10" plane through (0, 0, -44.45) normal (0, 0, -1) x (-1, 0, 0)
  line L0 (3.7395, 6.477) -> (7.479, 0)
  line L1 (7.479, 0) -> (3.7395, -6.477)
  line L2 (3.7395, -6.477) -> (-3.7395, -6.477)
  line L3 (-3.7395, -6.477) -> (-7.479, 0)
  line L4 (-7.479, 0) -> (-3.7395, 6.477)
  line L5 (-3.7395, 6.477) -> (3.7395, 6.477)
  point P0 (0, 0)
  point P1 (0, 0)
  dimension "d32" = 12.954
  constraints: 12 end point, 1 coincident, 1 horizontal, 13 other
  measures "d32" distance between parallel lines of L2 L5
extrude "Extrusion5" cut sketch "Sketch10" against normal through all
sketch "Sketch11" plane through (0, 0, -12.7) normal (0, 0, 1) x (1, 0, 0)
  line L0 (7.479, 0) -> (3.7395, 6.477) projected
  line L1 (3.7395, 6.477) -> (7.479, 0)
  line L2 (7.479, 0) -> (3.7395, -6.477)
  line L3 (3.7395, -6.477) -> (-3.7395, -6.477)
  line L4 (-3.7395, -6.477) -> (-7.479, 0)
  line L5 (-7.479, 0) -> (-3.7395, 6.477)
  line L6 (-3.7395, 6.477) -> (3.7395, 6.477)
  circle A0 centre (0, 0) radius 15.748
  constraints: 12 end point, 2 coincident, 1 centre point, 13 other
extrude "Extrusion6" add sketch "Sketch11" along normal blind 6.35
equation "\"d0\" = printedHexSize"
equation "\"d1\" = lengthOfHexExtrusion"
equation "\"hexSize\" = 12.7"
equation "\"slipFitOffset\" = 0"
equation "\"printedHexSize\" = hexSize - slipFitOffset"
equation "\"lengthOfHexExtrusion\" = 25.4"
equation "\"bushingSlipOffset\" = 0.381"
body "Solid1"
